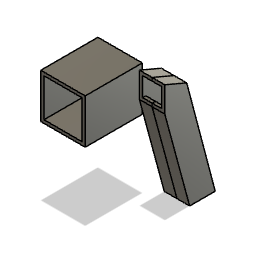
Contenedoryrampa (Autodesk Fusion 360 design; units mm, degrees)
Autodesk Fusion 360 part; units mm, degrees
sketch "Boceto1" plane through (0, 0, 0) normal (0, 0, 1) x (1, 0, 0)
  line L0 (-100, 100) -> (-100, 40)
  line L1 (-100, 40) -> (-40, 40)
  line L2 (-40, 40) -> (-40, 100)
  line L3 (-40, 100) -> (-100, 100)
  line L4 (-90, 90) -> (-90, 50)
  line L5 (-90, 50) -> (-50, 50)
  line L6 (-50, 50) -> (-50, 90)
  line L7 (-50, 90) -> (-90, 90)
  line L8 (-105, 35) -> (-35, 35)
  line L9 (-35, 35) -> (-35, 105)
  line L10 (-35, 105) -> (-105, 105)
  line L11 (-105, 105) -> (-105, 35)
  constraint vertical L0
  constraint perpendicular L0 L1
  constraint perpendicular L1 L2
  constraint perpendicular L0 L3
  constraint perpendicular L3 L4
  constraint perpendicular L4 L5
  constraint perpendicular L3 L6
  constraint perpendicular L4 L7
  constraint horizontal L8
  constraint perpendicular L8 L9
  constraint perpendicular L9 L10
  constraint perpendicular L8 L11
extrude "Extruir1" add sketch "Boceto1" along normal blind 10 contours L0 L1 L2 L3 | L8 L9 L10 L11 makes body 1
sketch "Boceto2" plane through (0, 0, 10) normal (0, 0, 1) x (1, 0, 0)
  line L0 (-90, 90) -> (-50, 90)
  line L1 (-50, 90) -> (-50, 50)
  line L2 (-50, 50) -> (-90, 50)
  line L3 (-90, 50) -> (-90, 90)
  line L4 (-105, 105) -> (-105, 35)
  line L5 (-105, 35) -> (-35, 35)
  line L6 (-35, 35) -> (-35, 105)
  line L7 (-35, 105) -> (-105, 105)
  line L8 (-100, 100) -> (-100, 40)
  line L9 (-100, 40) -> (-40, 40)
  line L10 (-40, 40) -> (-40, 100)
  line L11 (-40, 100) -> (-100, 100)
  constraint perpendicular L7 L8
  constraint perpendicular L8 L9
  constraint perpendicular L7 L10
  constraint perpendicular L8 L11
extrude "Extruir2" add sketch "Boceto2" along normal blind 80 contours L4 L5 L6 L7 bodies 1
sketch "Boceto3" plane through (0, 0, 0) normal (1, 0, 0) x (0, 0, -1)
sketch "Boceto4" plane through (0, 0, 0) normal (0, 0, -1) x (-1, 0, 0)
  line L0 (50, 90) -> (90, 90)
  line L1 (90, 90) -> (90, 50)
  line L2 (90, 50) -> (50, 50)
  line L3 (50, 50) -> (50, 90)
  line L4 (105, 35) -> (105, 105)
  line L5 (105, 105) -> (35, 105)
  line L6 (35, 105) -> (35, 35)
  line L7 (35, 35) -> (105, 35)
  line L8 (90, 50) -> (90, -135)
  line L9 (90, -135, 0) -> (90, -135, 50)
  line L10 (90, -135, 50) -> (90, 50, 0)
  dimension "d6" = 185
  dimension "d7" = 50
  constraint coincident L1.end L2.start
  constraint perpendicular L2 L8
  measures "d6" distance of L1.end L8.end
sketch "Boceto5" plane through (0, 0, 0) normal (0, 0, -1) x (-1, 0, 0)
  line L0 (50, 50) -> (50, -135)
  point P0 (50, 50)
  constraint coincident P0 L0.start
sketch "Boceto6" plane through (0, 0, 0) normal (0, 1, 0) x (1, 0, 0)
  line L0 (-50, 0) -> (-50, 50)
  line L1 (-50, 50) -> (-90, 50)
  constraint vertical L0
  constraint perpendicular L0 L1
sketch "Boceto7" plane through (-90, 0, 0) normal (-1, 0, 0) x (0, 0, 1)
sketch "Boceto8" plane through (0, 0, 0) normal (1, 0, 0) x (0, 0, -1)
  line L0 (50, -135, -90) -> (50, -135, -50)
  line L1 (50, -135, -50) -> (0, 50, -50)
  line L2 (50, -135, -90) -> (90, -135, -90)
  line L3 (90, -135, -90) -> (90, -135, -50)
  line L4 (50, -135, -50) -> (90, -135, -50)
  line L5 (0, 50, -50) -> (40, 50, -50)
  line L6 (90, -135, -90) -> (34.5742, 75.2911, -90)
  line L7 (90, -135, -50) -> (40, 50, -50)
  line L8 (0, 50, -90) -> (41.2401, 50, -90)
  line L9 (0, 90, -90) -> (34.5742, 75.2911, -90)
  line L10 (34.5742, 75.2911, -90) -> (34.5742, 75.2911, -50)
  line L11 (34.5742, 75.2911, -50) -> (40, 50, -50)
  line L12 (0, 90, -50) -> (34.5742, 75.2911, -50)
  line L13 (0, 90, -50) -> (0, 50, -50)
  line L14 (0, 90, -50) -> (0, 90, -90)
  line L15 (0, 90, -90) -> (0, 50, -90)
  line L16 (90, -135, -90) -> (50, -135, -90)
  line L17 (50, -135, -90) -> (0, 50, -90)
  line L18 (0, 90, -90) -> (0, 85, -90)
  line L19 (0, 55, -85) -> (0, 55, -55)
  line L20 (0, 55, -55) -> (0, 85, -55)
  line L21 (0, 85, -55) -> (0, 85, -85)
  line L22 (0, 85, -85) -> (0, 55, -85)
  line L23 (34.5742, 75.2911, -90) -> (34.5742, 75.2911, -85)
  line L24 (34.5742, 75.2911, -85) -> (29.5742, 75.2911, -85)
  line L25 (0, 85, -55) -> (0, 75.4843, -55)
  line L26 (0, 50, -50) -> (5, 50, -50)
  line L27 (5, 50, -50) -> (5, 50, -55)
  line L28 (5, 50, -55) -> (35, 50, -55)
  line L29 (5, 50, -55) -> (5, 50, -85)
  line L30 (34.5742, 75.2911, -50) -> (29.5742, 75.2911, -50)
  line L31 (0, 85, -55) -> (0, 85, -50)
  line L32 (29.5742, 75.2911, -50) -> (0, 85, -50)
  point P0 (50, -135)
  point P1 (0, 50)
  point P2 (0, 50)
  point P3 (0, 90)
  point P4 (0, 90)
  dimension "d8" = 40
  dimension "d9" = 40
  dimension "d10" = 40
  dimension "d18" = 5
  dimension "d20" = 30
  dimension "d21" = 30
  dimension "d22" = 5
  dimension "d24" = 5
  dimension "d27" = 5
  dimension "d28" = 5
  dimension "d29" = 30
  dimension "d30" = 30
  dimension "d31" = 5
  constraint coincident P2 P1
  constraint coincident P4 P3
sketch "Boceto8 (curves -90 mm off its plane)" plane through (-90, 0, 0) normal (1, 0, 0) x (0, 0, -1)
  line L0 (50, -135) -> (90, -135)
  line L1 (90, -135) -> (34.5742, 75.2911)
  line L2 (0, 50) -> (41.2401, 50)
  line L3 (0, 90) -> (34.5742, 75.2911)
  line L4 (0, 90) -> (0, 50)
  line L5 (90, -135) -> (50, -135)
  line L6 (50, -135) -> (0, 50)
  line L7 (0, 90) -> (0, 85)
extrude "Extruir5" add sketch "Boceto8 (curves -90 mm off its plane)" along normal blind 40 separate body makes body 2
shell "Vaciado3" thickness 5 removed faces 1 at (-76.6667, -135, -63.3333) on bodies 2
sketch "Boceto10" plane through (-90, 0, 0) normal (1, 0, 0) x (0, 0, -1)
  line L0 (35, 50, 35) -> (35, 50, 5)
  line L1 (35, 50, 5) -> (5, 50, 5)
  line L2 (0, 85, 5) -> (38.0789, 85, 5) construction
  line L3 (35, 50, 5) -> (75.1471, 50, 5) construction
  line L4 (33.6789, 55, 5) -> (29.0056, 72.6878, 5)
  line L5 (25.7526, 85, 5) -> (24.7446, 88.8152, 5)
  line L6 (0, 85, 5) -> (29.0056, 72.6878, 5)
  line L7 (35, 70.1434, 5) -> (35.0518, 70.1214, 5)
  line L8 (0, 55, 5) -> (33.6789, 55, 5)
  line L9 (29.5742, 70.5359, 5) -> (29.5742, 70.2911, 5)
  line L10 (33.6789, 55, 5) -> (0, 55, 5)
  line L11 (33.6789, 55, 5) -> (29.0056, 72.6878, 5)
  line L12 (0, 85, 5) -> (29.0056, 72.6878, 5)
  line L13 (0, 55, 5) -> (0, 85, 5)
  point P0 (29.5742, 75.2911)
  point P1 (0, 85)
  point P2 (35, 50)
  point P3 (5, 50)
  point P4 (0, 55)
  dimension "d35" = 5
  dimension "d36" = 30
  dimension "d37" = 23
  dimension "d38" = 104.8
sketch "Boceto10 (curves 5 mm off its plane)" plane through (-85, 0, 0) normal (1, 0, 0) x (0, 0, -1)
  line L0 (35, 50) -> (5, 50)
  line L1 (0, 85) -> (38.0789, 85) construction
  line L2 (35, 50) -> (75.1471, 50) construction
  line L3 (33.6789, 55) -> (29.0056, 72.6878)
  line L4 (25.7526, 85) -> (24.7446, 88.8152)
  line L5 (0, 85) -> (29.0056, 72.6878)
  line L6 (35, 70.1434) -> (35.0518, 70.1214)
  line L7 (0, 55) -> (33.6789, 55)
  line L8 (29.5742, 70.5359) -> (29.5742, 70.2911)
  line L9 (33.6789, 55) -> (0, 55)
  line L10 (33.6789, 55) -> (29.0056, 72.6878)
  line L11 (0, 85) -> (29.0056, 72.6878)
  line L12 (0, 55) -> (0, 85)
extrude "Extruir6" cut sketch "Boceto10 (curves 5 mm off its plane)" along normal blind 30 bodies 2
sketch "Boceto11" plane through (0, 0, 0) normal (0, 0, 1) x (1, 0, 0)
  line L0 (-35, 105) -> (-105, 105)
  line L1 (-70, 105) -> (-70, -135)
  line L2 (-90, -135, -50) -> (-50, -135, -50)
  constraint midpoint L0 L1.start
sketch "Boceto12" plane through (-90, 0, 0) normal (-1, 0, 0) x (0, 0, 1)
  line L0 (-34.5742, 75.2911) -> (-90, -135)
  line L1 (-90, -135) -> (-50, -135)
  line L2 (-50, -135) -> (0, 50)
  line L3 (0, 50) -> (0, 90)
  line L4 (0, 90) -> (-34.5742, 75.2911)
  line L5 (-50, -135) -> (-50, -95)
  line L6 (-90, -135) -> (-50, -135)
  line L7 (-50, -135) -> (-36.6386, -85.5629)
  line L8 (-90, -135) -> (-74.1517, -74.8698)
  line L9 (-50, -95) -> (-39.1789, -95)
  line L10 (-39.1789, -95) -> (-79.4573, -95)
  dimension "d41" = 40
  constraint vertical L5
  constraint coincident L1.end L2.start
  constraint coincident L0.end L1.start
  constraint coincident L2 L7.end
  constraint parallel L2 L7
  constraint coincident L0 L8.end
  constraint parallel L0 L8
  constraint perpendicular L5 L9
  constraint horizontal L10
  constraint coincident L8 L10.end
  measures "d41" distance of L1.end L5.end
extrude "Extruir7" cut sketch "Boceto12" against normal blind 40 contours L0 L1 L5 L6 L8 L10 | L2 L5 L7 L9 L10 bodies 2
sketch "Boceto13" plane through (0, 0, 0) normal (1, 0, 0) x (0, 0, -1)
move_body "Desplazar2" bodies 2 to x (1, 0, 0) y (0, 1, 0) z (0, 0, 1) at (70, 22.5, 19.5946)
split "Dividir1" by plane through (0, 0, 0) normal (1, 0, 0) bodies 2 makes body 3 at (20, 32.597, -18.4159)
sketch "Boceto14" plane through (0, 0, 0) normal (1, 0, 0) x (0, 0, -1)
sketch "Boceto15" plane through (0, 0, 0) normal (1, 0, 0) x (0, 0, -1)
  line L0 (9.411, 95.1878) -> (-19.5946, 107.5)
  line L1 (-19.5946, 107.5) -> (-19.5946, 112.5)
  line L2 (-19.5946, 112.5) -> (14.9796, 97.7911)
  line L3 (14.9796, 97.7911) -> (59.8627, -72.5)
  line L4 (59.8627, -72.5) -> (54.692, -72.5)
  line L5 (54.692, -72.5) -> (10.7688, 94.1488)
  line L6 (10.7688, 94.1488) -> (9.5484, 94.668)
  line L7 (9.5484, 94.668) -> (9.411, 95.1878)
  line L8 (-19.5946, 77.5) -> (-14.5946, 77.5)
  line L9 (-14.5946, 77.5) -> (-14.5946, 73.1638)
  line L10 (-14.5946, 73.1638) -> (24.774, -72.5)
  line L11 (24.774, -72.5) -> (19.5946, -72.5)
  line L12 (19.5946, -72.5) -> (-19.5946, 72.5)
  line L13 (-19.5946, 72.5) -> (-19.5946, 77.5)
extrude "Extruir3" [suppressed]
extrude "Extruir4" [suppressed]
sketch "Boceto9" plane through (0, -135, 0) normal (0, -1, 0) x (1, 0, 0)
  line L0 (-90, -50) -> (-90, -90)
  line L1 (-90, -90) -> (-50, -90)
  line L2 (-50, -90) -> (-50, -50)
  line L3 (-50, -50) -> (-90, -50)
  line L4 (-55, -54) -> (-55, -84)
  line L5 (-55, -84) -> (-85, -84)
  line L6 (-85, -84) -> (-85, -54)
  line L7 (-85, -54) -> (-55, -54)
  constraint perpendicular L3 L4
  constraint perpendicular L4 L5
  constraint perpendicular L5 L6
  constraint perpendicular L4 L7
shell "Vaciado1" [suppressed]
shell "Vaciado2" [suppressed]
move_body "Desplazar1" [suppressed]
